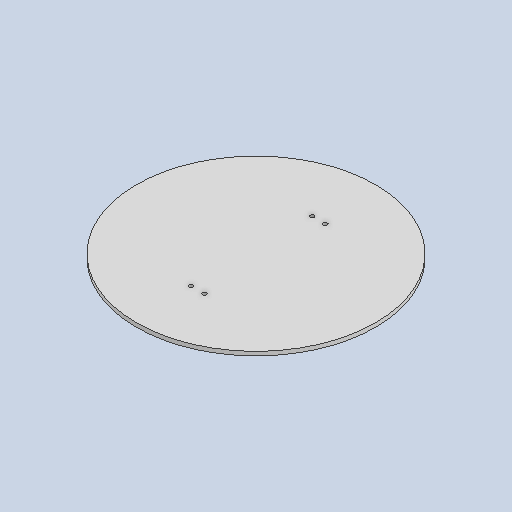
# Autodesk Inventor part: hiago_tampassl2
Saved by Autodesk Inventor 2023 (Build 270158000, 158)
## iProperties
Created: 2022-09-22
Part Number: hiago_tampassl2
Material: Generic
Document SubType Name: Modeling
Designer: hiago.sodre
Density: 1 g/cm^3
Appearance: Default
Author: hiago.sodre
Autodesk Inventor part; units mm, degrees
ref_plane "YZ Plane" through (0, 0, 0) normal (1, 0, 0) x (0, 1, 0)
ref_plane "XZ Plane" through (0, 0, 0) normal (0, 1, 0) x (-1, 0, 0)
ref_plane "XY Plane" through (0, 0, 0) normal (0, 0, 1) x (1, 0, 0)
sketch "Sketch1" plane through (0, 0, 0) normal (0, 1, 0) x (-1, 0, 0)
  circle A0 centre (0, 0) radius 90
  line L0 (0, 0) -> (3.3, 0) construction
  line L1 (3.3, 0) -> (3.3, 45.5) construction
  circle A1 centre (3.3, 45.5) radius 1.5
  line L2 (3.3, 45.5) -> (-6.7, 45.5) construction
  circle A2 centre (-6.7, 45.5) radius 1.5
  line L3 (3.3, 0) -> (3.3, -45.5) construction
  circle A3 centre (3.3, -45.5) radius 1.5
  line L4 (3.3, -45.5) -> (-6.7, -45.5) construction
  circle A4 centre (-6.7, -45.5) radius 1.5
  dimension "d0" = 180
  dimension "d1" = 3.3
  dimension "d2" = 45.5
  dimension "d3" = 3
  dimension "d4" = 10
  dimension "d5" = 3
  dimension "d6" = 45.5
  dimension "d7" = 3
  dimension "d8" = 10
  dimension "d9" = 3
  constraints: 10 end point, 5 centre point, 5 coincident, 3 horizontal, 1 perpendicular, 1 vertical
  measures "d0" diameter of A0
  measures "d1" distance of L0.start L0.end
  measures "d2" distance of L0.end L1.end
  measures "d3" diameter of A1
  measures "d4" distance of L2.start L2.end
  measures "d5" diameter of A2
  measures "d6" distance of L0.end L3.end
  measures "d7" diameter of A3
  measures "d8" distance of L4.start L4.end
  measures "d9" diameter of A4
extrude "Extrusion1" add sketch "Sketch1" along normal blind 3
body "Solid1"
